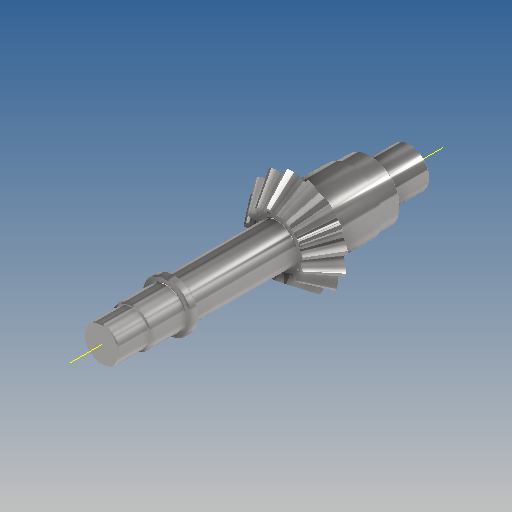
# Autodesk Inventor part: PWTR-0059
Saved by Autodesk Inventor 2021.1 (Build 251245000, 245)
## iProperties
CustomPartVersion: 1
Created: 2020-08-27
Part Number: PWTR-0059
Material: Steel, Mild
Document SubType Name: Modeling
Designer: alid
Categories: <?xml version="1.0" encoding="UTF-16"?> <MemberInstance><Categories><FamilyTemplate><FamilyTemplateParameter ValueType="xs:double" Id="1" ObjectReferenceKey="da_z" ObjectType="kUserParameterObject"/><FamilyTemplateParameter ValueType="xs:double" Id="2" ObjectReferenceKey="da_b" ObjectType="kUserParameterObject"/><FamilyTemplateParameter ValueType="xs:double" Id="3" ObjectReferenceKey="da_beta" ObjectType="kUserParameterObject"/><FamilyTemplateParameter ValueType="xs:double" Id="4" ObjectReferenceKey="da_dae" ObjectType="kUserParameterObject"/><FamilyTemplateParameter ValueType="xs:double" Id="5" ObjectReferenceKey="da_ve" ObjectType="kUserParameterObject"/><FamilyTemplateParameter ValueType="xs:double" Id="6" ObjectReferenceKey="da_omega" ObjectType="kUserParameterObject"/><FamilyTemplateParameter ValueType="xs:string" Id="7" ObjectReferenceKey="EAIAABAAAAAAHwAAAAAAAIAAAAAAAAAA" ObjectType="83914240" SubObjectId="SurfaceGeometry"/></FamilyTemplate><ParamToTemplateMap><ParamToTemplate CategoryParameter="//CategoryParameter[@InternalName='046C89C9-8512-4d59-83FE-43B91F4F132A']" TemplateParameter="1"/><ParamToTemplate CategoryParameter="//CategoryParameter[@InternalName='2552DF32-E462-4b46-AEBF-C6C7768E72AC']" TemplateParameter="2"/><ParamToTemplate CategoryParameter="//CategoryParameter[@InternalName='C9EE641D-15FC-4fae-A226-E94C4372FDD7']" TemplateParameter="3"/><ParamToTemplate><ParamToTemplate CategoryParameter="//CategoryParameter[@InternalName='00B6519A-459B-49c7-AD84-2E56D39A5744']" ConstantValue="-0.000000"/></ParamToTemplate><ParamToTemplate><ParamToTemplate CategoryParameter="//CategoryParameter[@InternalName='04B31F0E-C7A6-4894-AA32-9629BEFACF47']" ConstantValue="1.000000"/></ParamToTemplate><ParamToTemplate><ParamToTemplate CategoryParameter="//CategoryParameter[@InternalName='43CBEC2E-7847-49e7-A936-2F7889FCB2D9']" ConstantValue="0.200000"/></ParamToTemplate><ParamToTemplate><ParamToTemplate CategoryParameter="//CategoryParameter[@InternalName='B1EFC894-105D-4ebd-86BF-FA20ED196853']" ConstantValue="0.266800"/></ParamToTemplate><ParamToTemplate><ParamToTemplate CategoryParameter="//CategoryParameter[@InternalName='51175063-3D10-4879-93E8-6246FE8B403D']" ConstantValue="2060000000.000000"/></ParamToTemplate><ParamToTemplate><ParamToTemplate CategoryParameter="//CategoryParameter[@InternalName='A3A52E27-4454-46a9-B0BD-C932399B70AF']" ConstantValue="0.300000"/></ParamToTemplate><ParamToTemplate CategoryParameter="//CategoryParameter[@InternalName='2A200944-5A8C-41ca-B96E-8520D2E510F1']" TemplateParameter="4"/><ParamToTemplate><ParamToTemplate CategoryParameter="//CategoryParameter[@InternalName='1A637F62-92C8-44bc-B81F-10802510B579']" ConstantValue="3.010702"/></ParamToTemplate><ParamToTemplate CategoryParameter="//CategoryParameter[@InternalName='B52DD4BE-6863-48fb-BF58-89EF6F9EC65C']" TemplateParameter="5"/><ParamToTemplate><ParamToTemplate CategoryParameter="//CategoryParameter[@InternalName='3956BFF2-84D2-457d-93C2-9B0613DEBA67']" ConstantValue="1.977690"/></ParamToTemplate><ParamToTemplate CategoryParameter="//CategoryParameter[@InternalName='739CFA02-461B-4bf8-8049-181FCAD8B28F']" TemplateParameter="6"/><ParamToTemplate><ParamToTemplate CategoryParameter="//CategoryParameter[@InternalName='A27E999F-E2CE-4481-8A2A-EBF499C4C3C5']" ConstantValue="-0.000000"/></ParamToTemplate><ParamToTemplate><ParamToTemplate CategoryParameter="//CategoryParameter[@InternalName='9E1B4470-B2D3-4ff1-B813-535BB4CDF51A']" ConstantValue="3520000.000000"/></ParamToTemplate><ParamToTemplate><ParamToTemplate CategoryParameter="//CategoryParameter[@InternalName='F8452263-BFF6-458c-9FB1-07C4B99E95CD']" ConstantValue="11400000.000000"/></ParamToTemplate><ParamToTemplate><ParamToTemplate CategoryParameter="//CategoryParameter[@InternalName='3E3BB259-FD49-497f-8171-6EBC954A3479']" ConstantValue="2.000000"/></ParamToTemplate><ParamToTemplate CategoryParameter="//CategoryParameter[@InternalName='27C3BAF2-7550-4e4b-AE2C-0DB134B7D9B7']" TemplateParameter="7"/></ParamToTemplateMap><Category DisplayName="Gear" InternalName="DC85795E-93AB-48d5-8EEE-5A27447B64BD" Mnemonic="Gear"><CategoryParameter DisplayName="z" InternalName="046C89C9-8512-4d59-83FE-43B91F4F132A" Mnemonic="z"/><CategoryParameter DisplayName="b" InternalName="2552DF32-E462-4b46-AEBF-C6C7768E72AC" Mnemonic="b"/><CategoryParameter DisplayName="||b|" InternalName="C9EE641D-15FC-4fae-A226-E94C4372FDD7" Mnemonic="beta"/><CategoryParameter DisplayName="x" InternalName="00B6519A-459B-49c7-AD84-2E56D39A5744" Mnemonic="x"/><CategoryParameter DisplayName="a*" InternalName="04B31F0E-C7A6-4894-AA32-9629BEFACF47" Mnemonic="a"/><CategoryParameter DisplayName="c*" InternalName="43CBEC2E-7847-49e7-A936-2F7889FCB2D9" Mnemonic="c"/><CategoryParameter DisplayName="r|.f|*" InternalName="B1EFC894-105D-4ebd-86BF-FA20ED196853" Mnemonic="rf"/><CategoryParameter DisplayName="E" InternalName="51175063-3D10-4879-93E8-6246FE8B403D" Mnemonic="E"/><CategoryParameter DisplayName="||m|" InternalName="A3A52E27-4454-46a9-B0BD-C932399B70AF" Mnemonic="mi"/><Category DisplayName="BevelGear" InternalName="0C98F69A-0C2B-4791-B2FE-7691BB227E77" Mnemonic="BevelGear"><CategoryParameter DisplayName="d|.ae|" InternalName="2A200944-5A8C-41ca-B96E-8520D2E510F1" Mnemonic="dae"/><CategoryParameter DisplayName="d|.ai|" InternalName="1A637F62-92C8-44bc-B81F-10802510B579" Mnemonic="dai"/><CategoryParameter DisplayName="A|.e|" InternalName="B52DD4BE-6863-48fb-BF58-89EF6F9EC65C" Mnemonic="ve"/><CategoryParameter DisplayName="A|.i|" InternalName="3956BFF2-84D2-457d-93C2-9B0613DEBA67" Mnemonic="vi"/><CategoryParameter DisplayName="||S|" InternalName="739CFA02-461B-4bf8-8049-181FCAD8B28F" Mnemonic="omega"/><CategoryParameter DisplayName="x|.t|" InternalName="A27E999F-E2CE-4481-8A2A-EBF499C4C3C5" Mnemonic="xt"/><CategoryParameter DisplayName="||s||.Flim|" InternalName="9E1B4470-B2D3-4ff1-B813-535BB4CDF51A" Mnemonic="sFlim"/><CategoryParameter DisplayName="||s||.Hlim|" InternalName="F8452263-BFF6-458c-9FB1-07C4B99E95CD" Mnemonic="sHlim"/><CategoryParameter DisplayName="type" InternalName="3E3BB259-FD49-497f-8171-6EBC954A3479" Mnemonic="type"/><CategoryParameter DisplayName="PitchDiameter" InternalName="27C3BAF2-7550-4e4b-AE2C-0DB134B7D9B7" Mnemonic="IDS_PITCHDIAM"/></Category></Category></Categories></MemberInstance>
Mass: 60.9118 g
Surface Area: 34.3074 cm^2
Volume: 7.7496 cm^3
Density: 7.86 g/cm^3
Appearance: Steel - Polished
Description: Bevel Gear Drive Shaft
Author: alid
Revision Number: A
Autodesk Inventor part; units mm, degrees
ref_plane "Mesh Plane2" through (0, 0, 0) normal (0.9781476, 0.2079117, 0) x (0, 0, 1)
sketch "Teeth Body Sketch" plane through (0, 0, 0) normal (1, 0, 0) x (0, 1, 0)
  line L0 (0, 0) -> (19.484602, -36.466564) construction
  line L1 (19.484602, -36.466564) -> (25.012832, -32.861197)
  line L2 (25.012832, -32.861197) -> (0, 0) construction
  line L3 (22.5, -34.5) -> (0, 0) construction
  line L4 (11.726447, -21.946726) -> (15.05351, -19.776903)
  line L5 (19.484602, -36.466564) -> (11.726447, -21.946726)
  line L6 (25.012832, -32.861197) -> (15.05351, -19.776903)
  line L7 (0, -28.011419) -> (0, 4.66857)
  line L8 (0, -34.5) -> (25.012832, -34.5) construction
  dimension "d0" = 45
  dimension "d1" = 38.9692
  dimension "d2" = 50.02566
  dimension "d3" = 16.4
  dimension "d4" = 32.8612
  constraints: 16 end point, 4 point on line, 3 perpendicular, 2 collinear, 1 horizontal alignment, 1 vertical alignment
  measures "d0" diameter of L3.start L7
  measures "d1" diameter of L0.end L7
  measures "d2" diameter of L1.end L7
  measures "d3" distance between parallel lines of L1 L4
  measures "d4" vertical distance of L1.end L0.start
revolve "Teeth Body" add sketch "Teeth Body Sketch" angle 360 about axis through (0, 0, 0) along (0, 0, 1)
ref_plane "Tooth Plane" through (0, 22.5, -34.5) normal (0, -0.5462678, 0.8376106) x (1, 0, 0)
sketch "Start Sketch" plane through (0, 22.5, -34.5) normal (0, -0.5462678, 0.8376106) x (1, 0, 0)
  line L0 (0, -29.426237) -> (0, 10.605622)
  arc A0 (-1.344185, -4.392) -> (-6.54153, 4.300823) centre (-11.534443, -4.584516) ccw
  arc A1 (6.54153, 4.300823) -> (1.344185, -4.392) centre (11.534443, -4.584516) ccw
  line L1 (-1.344185, -4.392) -> (1.344185, -4.392)
  arc A2 (6.54153, 4.300823) -> (-6.54153, 4.300823) centre (0, -26.862124) ccw
  dimension "d7" = 10.19208
  dimension "d8" = 11.53444
  dimension "d9" = 22.27761
  dimension "d57" = 31.84212
  dimension "d58" = 22.47012
  constraints: 6 point on circle, 3 centre point, 3 symmetric about line, 2 end point, 1 coincident, 1 perpendicular, 1 other
  measures "d7" radius of A0
  measures "d8" horizontal distance of point (0, -26.862) A0.centre
  measures "d9" vertical distance of point (0, -26.862) A0.centre
  measures "d57" radius of A2
  measures "d58" distance from line of A2.centre L1
sketch "End Sketch" plane through (0, 13.36094, -20.486775) normal (0, -0.5462678, 0.8376106) x (1, 0, 0)
  line L0 (0, -17.375975) -> (0, 6.262541)
  arc A0 (-0.798203, -2.608055) -> (-3.884489, 2.553913) centre (-6.849378, -2.722375) ccw
  arc A1 (3.884489, 2.553913) -> (0.798203, -2.608055) centre (6.849378, -2.722375) ccw
  line L1 (-0.798203, -2.608055) -> (0.798203, -2.608055)
  arc A2 (3.884489, 2.553913) -> (-3.884489, 2.553913) centre (0, -15.951255) ccw
  dimension "d12" = 6.05225
  dimension "d15" = 6.84938
  dimension "d16" = 13.22888
  dimension "d59" = 18.90848
  dimension "d60" = 13.3432
  constraints: 6 point on circle, 3 centre point, 3 symmetric about line, 2 end point, 1 coincident, 1 other
  measures "d12" radius of A0
  measures "d15" horizontal distance of A0.centre point (0, -15.951)
  measures "d16" vertical distance of A0.centre point (0, -15.951)
  measures "d59" radius of A2
  measures "d60" distance from line of A2.centre L1
loft "Loft" cut profiles "Start Sketch", "End Sketch"
pattern_circular "Circular Pattern" count 15 over 360 about axis through (0, 0, 0) along (0, 0, 1) of "Loft"
ref_plane "End Plane" through (0, 13.36094, -20.486775) normal (0, -0.5462678, 0.8376106) x (1, 0, 0)
sketch3d "3D Sketch Right"
ref_plane "End Plane Right" through (-4.813083, 12.463906, -20.486775) normal (0.196785, -0.5095922, 0.8376106) x (0.9328615, 0.3602353, 0)
sketch "End Sketch Right" plane through (-4.813083, 12.463906, -20.486775) normal (0.196785, -0.5095922, 0.8376106) x (0.9328615, 0.3602353, 0)
  arc A0 (-0.798203, -2.608055) -> (-3.884489, 2.553913) centre (-6.849378, -2.722375) ccw
  line L0 (0, -24.563202) -> (0, 11.497558)
  arc A1 (3.884489, 2.553913) -> (0.798203, -2.608055) centre (6.849378, -2.722375) ccw
  line L1 (-0.798203, -2.608055) -> (0.798203, -2.608055)
  arc A2 (3.884489, 2.553913) -> (-3.884489, 2.553913) centre (0, -15.951255) ccw
  dimension "d70" = 6.84938
  dimension "d71" = 13.22888
  dimension "d72" = 6.05225
  dimension "d73" = 13.3432
  dimension "d74" = 18.90848
  constraints: 6 point on circle, 3 centre point, 3 symmetric about line, 2 end point, 1 coincident, 1 perpendicular, 1 other
  measures "d70" horizontal distance of A2.centre A0.centre
  measures "d71" vertical distance of point (0, -15.951) A0.centre
  measures "d72" radius of A0
  measures "d73" distance from line of point (0, -15.951) L1
  measures "d74" radius of A2
feature "Loft Right" [suppressed]
pattern_circular "Circular Pattern Right" [suppressed]
sketch3d "3D Sketch Left"
ref_plane "End Plane Left" through (4.636742, 12.463906, -20.427443) normal (-0.1902272, -0.5113448, 0.8380573) x (0.9372462, -0.3486683, 0)
sketch "End Sketch Left" plane through (4.636742, 12.463906, -20.427443) normal (-0.1902272, -0.5113448, 0.8380573) x (0.9372462, -0.3486683, 0)
  line L0 (0, -29.996203) -> (0, 16.149028)
  arc A0 (-0.798203, -2.588037) -> (-3.884489, 2.573932) centre (-6.849378, -2.702356) ccw
  arc A1 (3.884489, 2.573932) -> (0.798203, -2.588037) centre (6.849378, -2.702356) ccw
  line L1 (-0.798203, -2.588037) -> (0.798203, -2.588037)
  ellipse E0 centre (0, -10.789926) end of major axis (15.05351, -10.789926) minor radius 12.615704
  arc A2 (3.884489, 2.573932) -> (-3.884489, 2.573932) centre (0, -15.931236) ccw
  dimension "d56" = 12.6157
  dimension "d30" = 6.05225
  dimension "d31" = 6.84938
  dimension "d32" = 13.22888
  dimension "d61" = 18.90848
  dimension "d62" = 13.3432
  constraints: 6 point on circle, 3 centre point, 3 symmetric about line, 2 end point, 1 coincident, 2 other
  measures "d30" radius of A0
  measures "d31" horizontal distance of point (0, -15.931) A0.centre
  measures "d32" vertical distance of A0.centre point (0, -15.931)
  measures "d61" radius of A2
  measures "d62" distance from line of point (0, -15.931) L1
feature "Loft Left" [suppressed]
pattern_circular "Circular Pattern Left" [suppressed]
sketch "Body Sketch" plane through (0, 0, 0) normal (1, 0, 0) x (0, 1, 0)
  line L0 (0, -25.199566) -> (0, -12.202544)
  line L1 (19.484602, -36.466564) -> (11.726447, -21.946726)
  line L2 (11.726447, -21.946726) -> (0, -21.946726)
  line L3 (19.484602, -36.466564) -> (0, -36.466564)
  constraints: 4 end point, 2 perpendicular, 2 point on line
sketch "Body Sketch outline for Fix Body" plane through (0, 0, 0) normal (1, 0, 0) x (0, 1, 0)
  line L0 (0, -36.466564) -> (19.484602, -36.466564)
  line L1 (0, -21.946726) -> (0, -36.466564)
  line L2 (11.726447, -21.946726) -> (0, -21.946726)
  line L3 (19.484602, -36.466564) -> (11.726447, -21.946726)
revolve "Fix Body" add sketch "Body Sketch outline for Fix Body" angle 360 about axis through (0, 0, 0) along (0, 0, 1)
sketch "Sketch6" plane through (0, 0, 0) normal (1, 0, 0) x (0, 1, 0)
  line L0 (22.5, -34.5) -> (0, 0) projected
  line L1 (0, -25.2) -> (0, 4.2) projected
surface revolve "Pitch Diameter" sketch "Sketch6" angle 360 about axis through (0, 0, 0) along (0, 0, 1) shown no curves L0
sketch "Sketch9" plane through (0, 0, 0) normal (1, 0, 0) x (0, 1, 0)
  line L0 (0, 67.533436) -> (0, -89.466564)
  line L1 (0, -89.466564) -> (10, -89.466564)
  line L2 (10, -89.466564) -> (10, -69.466564)
  line L3 (10, -69.466564) -> (16, -69.466564)
  line L4 (4.688649, -36.466564) -> (7.323037, -36.466564)
  line L5 (16, -69.466564) -> (16, -36.466564)
  line L6 (16, -36.466564) -> (0, -36.466564)
  line L7 (10, -36.466564) -> (10, 30.533436)
  line L8 (10, 30.533436) -> (12.5, 30.533436)
  line L9 (12.5, 30.533436) -> (12.5, 34.533436)
  line L10 (12.5, 34.533436) -> (10, 34.533436)
  line L11 (10, 34.533436) -> (10, 52.533436)
  line L12 (10, 52.533436) -> (9, 52.533436)
  line L13 (9, 52.533436) -> (9, 67.533436)
  line L14 (9, 67.533436) -> (0, 67.533436)
  line L15 (15, -69.466564) -> (15, -59.466564)
  line L16 (15, -59.466564) -> (16, -59.466564)
  point P0 (0, 0)
  dimension "d100" = 20
  dimension "d101" = 32
  dimension "d104" = 25
  dimension "d105" = 4
  dimension "d106" = 67
  dimension "d110" = 33
  dimension "d111" = 20
  dimension "d112" = 18
  dimension "d113" = 15
  dimension "d114" = 20
  dimension "d115" = 18
  dimension "d120" = 10
  dimension "d121" = 30
  constraints: 32 end point, 11 perpendicular, 7 point on line, 5 vertical
  measures "d100" diameter of L2 L0
  measures "d101" diameter of L5 L0
  measures "d104" diameter of L9 L0
  measures "d105" distance of L8.end L9.end
  measures "d106" distance of L7.start L7.end
  measures "d110" distance between parallel lines of L3 L6
  measures "d111" distance of L1.end L2.end
  measures "d112" distance of L10.end L11.end
  measures "d113" distance of L12.end L13.end
  measures "d114" diameter of L11 L0
  measures "d115" diameter of L13 L0
  measures "d120" distance of L15.start L15.end
  measures "d121" diameter of L15 L0
revolve "Revolution3" add sketch "Sketch9" angle 360 about axis through (0, 0, 67.533436) along (0, 0, -1) contours L14 L13 L12 L11 L10 L9 L8 L7 L6 L4 L0 | L6 L4 L5 L16 L15 L3 L2 L1 L0
sketch "Sketch10" plane through (0, 0, -89.466564) normal (0, 0, -1) x (-1, 0, 0)
  circle A0 centre (0, 0) radius 10 projected
  point P0 (0, 0)
  constraints: 1 coincident
hole "Hole1" at (0, 0, -89.466564) direction (0, 0, 1) diameter 4.917 depth 17.1 tip angle 118 thread size "M6x1" class "6H" standard "ISO Metric profile"
chamfer "Chamfer1" distance 0.5 angle 45 7 edges at (0, -10, 52.5334) (0, -9, 67.5334) (0, -12.5, 34.5334) (0, -12.5, 30.5334) (0, -10, -89.4666) (0, -16, -59.4666) (0, -15, -69.4666)
fillet "Fillet1" radius 0.5 5 edges at (0, -10, 34.5334) (0, -10, 30.5334) (0, -10, -21.9467) (0, -16, -36.4666) (0, -10, -69.4666)
equation "\"d0\" = da_de"
equation "\"d1\" = da_dfe"
equation "\"d2\" = da_dae"
equation "\"d3\" = da_b"
equation "\"d4\" = da_ve"
equation "\"d7\" = fd_rr"
equation "\"d8\" = fd_x"
equation "\"d9\" = fd_y"
equation "\"d57\" = 0.5 * fd_dva + 0.3 * da_he"
equation "\"d58\" = 0.5 * fd_dva - 1.12 * da_he"
equation "\"da_teethtype\" = 0"
equation "\"da_b\" = 16.4"
equation "\"da_de\" = 45"
equation "\"da_dae\" = 50.02566"
equation "\"da_dfe\" = 38.9692"
equation "\"da_le\" = 41.18859"
equation "\"da_omega\" = 90deg"
equation "\"da_beta\" = 0"
equation "\"da_delta\" = 33.111342deg"
equation "\"da_alpha\" = 20deg"
equation "\"da_he\" = 6.6"
equation "\"da_ve\" = 32.8612"
equation "\"da_zv\" = 17.908083"
equation "\"fd_loft\" = da_b + 0.05 * da_he"
equation "\"fd_x\" = fd_x1 + fd_x2"
equation "\"fd_y\" = fd_y1 - fd_y2"
equation "\"fd_dd\" = fd_dva - 0.8 * da_he"
equation "\"da_dvw\" = 53.72425"
equation "\"d11\" = fd_loft"
equation "\"da_dm\" = 36.04121"
equation "\"da_x\" = 0"
equation "\"da_m\" = 3"
equation "\"d50\" = da_omega"
equation "\"fd_rr\" = 10.192076"
equation "\"fd_dva\" = 59.724249"
equation "\"fd_x1\" = 2.379252"
equation "\"fd_x2\" = 9.155191"
equation "\"fd_y1\" = 26.756548"
equation "\"fd_y2\" = 4.47894"
body "Solid1"
body "Srf1"
